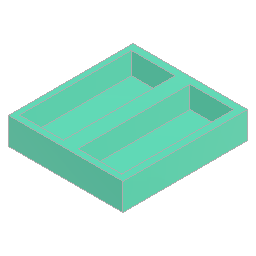
Eraser-Carrier (Autodesk Fusion 360 design; units mm, degrees)
Autodesk Fusion 360 part; units mm, degrees
sketch "Sketch1" plane through (0, 0, 32.475) normal (0, 0, 1) x (-1, 0, 0)
  line L0 (-197.1, 152.972) -> (-197.1, 218.046)
  line L1 (-197.1, 218.046) -> (-171.65, 218.046)
  line L2 (-171.65, 218.046) -> (-171.65, 152.972)
  line L3 (-171.65, 152.972) -> (-197.1, 152.972)
  line L4 (-137.55, 152.972) -> (-163, 152.972)
  line L5 (-163, 152.972) -> (-163, 218.046)
  line L6 (-163, 218.046) -> (-137.55, 218.046)
  line L7 (-137.55, 218.046) -> (-137.55, 152.972)
  line L8 (-201.1, 221.472) -> (-201.1, 148.972)
  line L9 (-201.1, 148.972) -> (-134.55, 148.972)
  line L10 (-134.55, 148.972) -> (-134.55, 221.472)
  line L11 (-134.55, 221.472) -> (-201.1, 221.472)
extrude "Extrude1" add sketch "Sketch1" along normal blind 3 contours L0 L1 L2 L3 | L4 L5 L6 L7 | L8 L9 L10 L11
extrude "Extrude2" add sketch "Sketch1" along normal up to surface (15.7 mm away)
